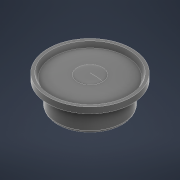
# Autodesk Inventor part: Speaker_28mm
Saved by Autodesk Inventor 2022 (Build 260153000, 153)
## iProperties
Created: 2024-05-10
Part Number: Speaker_28mm
Material: Generic
Document SubType Name: Modeling
Designer: jo_ki
Density: 1 g/cm^3
Appearance: Smooth - Black
Author: jo_ki
Autodesk Inventor part; units mm, degrees
ref_plane "YZ Plane" through (0, 0, 0) normal (1, 0, 0) x (0, 1, 0)
ref_plane "XZ Plane" through (0, 0, 0) normal (0, 1, 0) x (-1, 0, 0)
ref_plane "XY Plane" through (0, 0, 0) normal (0, 0, 1) x (1, 0, 0)
sketch "Sketch1" plane through (0, 0, 0) normal (0, 0, 1) x (1, 0, 0)
  line L0 (-7.8193, 0) -> (17.6366, 0) projected
  line L1 (0, -62.7697) -> (0, 10.4616) projected
  line L2 (0, 0) -> (14, 0)
  line L3 (14, 0) -> (14, -2)
  line L4 (14, -2) -> (0, -2)
  line L5 (0, -2) -> (0, 0)
  line L6 (0, -2) -> (11, -2)
  line L7 (11, -2) -> (11, -10)
  line L8 (11, -10) -> (0, -10)
  line L9 (0, -10) -> (0, -2)
  ellipse E0 centre (0, -0.5609) end of major axis (4.1828, -0.5609) minor radius 0.5609
  arc A0 (12.2031, -1.4564) -> (4.1828, -0.5609) centre (2.4654, -52.3081) ccw
  line L10 (12.2031, -1.4564) -> (13.04, 0)
  point P0 (0, -10)
  dimension "d1" = 28
  dimension "d2" = 10
  dimension "d3" = 2
  dimension "d5" = 3
  constraints: 18 end point, 4 parallel, 3 horizontal, 2 perpendicular, 2 point on circle, 2 point on line, 1 centre point, 1 vertical, 3 other
  measures "d1" diameter of L3 L1
  measures "d2" distance between parallel lines of L8 L0
  measures "d3" distance between parallel lines of L0 L4
  measures "d5" distance between parallel lines of L3 L7
revolve "Revolution1" add sketch "Sketch1" angle 360 about axis through (0, -10, 0) along (0, 1, 0) picked at (0.7846, -0.4063) contours E0 L1 | L0 L3 L4 L1 E0 A0 L10 | L4 L7 L8 L1
fillet "Fillet1" radius 1 1 edges at (-11, -10, 0)
body "Solid1"
